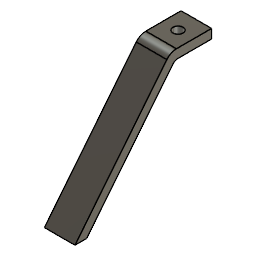
Tope caida_ (Autodesk Fusion 360 design; units mm, degrees)
Autodesk Fusion 360 part; units mm, degrees
note: some values were not read from the file. Set by a fixed rule: which sketch regions a step uses.
sketch "Boceto1" plane through (0, 0, 0) normal (1, 0, 0) x (0, 1, 0)
  line L0 (0, 36) -> (12, 36)
  line L1 (12, 36) -> (12, 39)
  line L2 (12, 39) -> (0, 39)
  line L3 (0, 36) -> (-28.8001, -0.0001)
  line L4 (-1.4419, 39) -> (0, 39)
  line L5 (-28.8001, -0.0001) -> (-32.6419, -0.0001)
  line L6 (-32.6419, -0.0001) -> (-1.4419, 39)
  dimension "d3" = 12
  dimension "d4" = 3
  dimension "d14" = 36
  constraint perpendicular L0 L1
  constraint perpendicular L1 L2
  constraint parallel L2 L4
  measures "d3" distance of L0.start L0.end
  measures "d4" distance of L0.end L1.end
  measures "d14" distance of origin L0.start
extrude "Extruir1" add sketch "Boceto1" against normal blind 10
sketch "Boceto2" plane through (0, 0, 39) normal (0, 0, 1) x (-1, 0, 0)
  line L0 (0, 1.4419) -> (0, -12)
  line L1 (0, -12) -> (10, -12)
  line L2 (10, -12) -> (10, 1.4419)
  circle A0 centre (5, -6) radius 1.65
  line L3 (10, 1.4419) -> (0, 1.4419)
  dimension "d7" = 3.3
  measures "d7" diameter of A0
extrude "Extruir2" cut sketch "Boceto2" against normal blind 3 contours A0
fillet "Empalme1" radius 4 1 edges at (-5, -1.4419, 39)
fillet "Empalme2" radius 2 1 edges at (-5, 0, 36)
